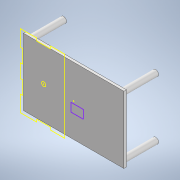
# Autodesk Inventor part: table top
Saved by Autodesk Inventor 2020 (Build 240168000, 168)
## iProperties
Created: 2022-02-14
Part Number: table top
Material: Generic
Document SubType Name: Modeling
Designer: rwte
Density: 1 g/cm^3
Appearance: Default
Author: rwte
Autodesk Inventor part; units mm, degrees
ref_plane "YZ Plane" through (0, 0, 0) normal (1, 0, 0) x (0, 1, 0)
ref_plane "XZ Plane" through (0, 0, 0) normal (0, 1, 0) x (-1, 0, 0)
ref_plane "XY Plane" through (0, 0, 0) normal (0, 0, 1) x (1, 0, 0)
sketch "Sketch1" plane through (0, 0, 0) normal (0, 0, 1) x (1, 0, 0)
  line L0 (-50, -30) -> (50, -30) construction
  line L1 (50, -30) -> (50, 30) construction
  line L2 (50, 30) -> (-50, 30) construction
  line L3 (-50, 30) -> (-50, -30) construction
  line L4 (-50, -30) -> (50, 30) construction
  line L5 (50, -30) -> (-50, 30) construction
  line L6 (-60, -40) -> (60, -40)
  line L7 (60, -40) -> (60, 40)
  line L8 (60, 40) -> (-60, 40)
  line L9 (-60, 40) -> (-60, -40)
  line L10 (-60, -40) -> (60, 40)
  line L11 (60, -40) -> (-60, 40)
  point P0 (0, 0)
  dimension "d0" = 60
  dimension "d1" = 100
  dimension "d2" = 10
  dimension "d3" = 10
  constraints: 24 end point, 4 midpoint, 4 parallel, 2 horizontal, 2 perpendicular
  measures "d0" distance of L0.end L1.end
  measures "d1" distance of L1.end L2.end
  measures "d2" distance between parallel lines of L7 L1
  measures "d3" horizontal distance of L7.end L1.end
extrude "Extrusion1" add sketch "Sketch1" along normal blind 3
sketch "Sketch2" plane through (0, 0, 0) normal (0, 0, -1) x (-1, 0, 0)
  line L0 (50, -30) -> (50, 30) construction
  line L1 (50, 30) -> (-50, 30) construction
  line L2 (-50, 30) -> (-50, -30) construction
  line L3 (-50, -30) -> (50, -30) construction
  line L4 (50, -30) -> (-50, 30) construction
  line L5 (50, 30) -> (-50, -30) construction
  line L6 (60, -40) -> (-60, -40) construction
  line L7 (-50, -30) -> (-60, -30) construction
  line L8 (-60, -30) -> (-60, -40) construction
  line L9 (-60, -40) -> (-50, -40) construction
  line L10 (-50, -40) -> (-50, -30) construction
  line L11 (-60, 40) -> (60, 40) construction
  line L12 (-50, 30) -> (-60, 30) construction
  line L13 (-60, 30) -> (-60, 40) construction
  line L14 (-60, 40) -> (-50, 40) construction
  line L15 (-50, 40) -> (-50, 30) construction
  line L16 (50, 30) -> (60, 30) construction
  line L17 (60, 30) -> (60, 40) construction
  line L18 (60, 40) -> (50, 40) construction
  line L19 (50, 40) -> (50, 30) construction
  line L20 (60, 40) -> (60, -40) construction
  line L21 (60, -40) -> (50, -40) construction
  line L22 (50, -40) -> (50, -30) construction
  line L23 (50, -30) -> (60, -30) construction
  line L24 (60, -30) -> (60, -40) construction
  circle A0 centre (-55, -35) radius 3.5
  circle A1 centre (-55, 35) radius 3.5
  circle A2 centre (55, -35) radius 3.5
  circle A3 centre (55, 35) radius 3.5
  line L25 (-55, -35) -> (55, -35) construction
  line L26 (55, -35) -> (55, 35) construction
  line L27 (55, 35) -> (-55, 35) construction
  line L28 (-55, 35) -> (-55, -35) construction
  line L29 (-55, -35) -> (55, 35) construction
  line L30 (55, -35) -> (-55, 35) construction
  line L31 (-60, -40) -> (-60, 40) construction
  point P0 (0, 0)
  dimension "d6" = 60
  dimension "d7" = 100
  dimension "d8" = 7
  dimension "d9" = 7
  dimension "d10" = 7
  dimension "d11" = 7
  dimension "d12" = 5
  dimension "d13" = 5
  constraints: 56 end point, 12 parallel, 6 perpendicular, 5 horizontal, 4 centre point, 4 midpoint, 3 coincident, 1 vertical
  measures "d6" distance of L1.end L2.end
  measures "d7" distance of L0.end L1.end
  measures "d8" diameter of A0
  measures "d9" diameter of A1
  measures "d10" diameter of A2
  measures "d11" diameter of A3
  measures "d12" distance between parallel lines of L31 L28
  measures "d13" distance between parallel lines of L6 L25
extrude "Extrusion2" add sketch "Sketch2" along normal blind 40
equation "\"d3\" = d2"
equation "\"d6\" = d0"
equation "\"d7\" = d1"
equation "\"d12\" = 0.5 * d2"
equation "\"d13\" = d12"
body "Solid1"
